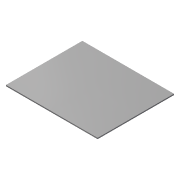
# Autodesk Inventor part: Деталь141
Saved by Autodesk Inventor 2017 (Build 210142000, 142)
## iProperties
Created: 2018-07-05
Part Number: Деталь141
Material: Сталь
Document SubType Name: Sheet Metal
Designer: Евтушенко
Mass: 6256.27 g
Surface Area: 5387.28 cm^2
Volume: 796.978 cm^3
Density: 7.85 g/cm^3
Sheet Metal Rule: ЧЗСК 1,5 мм
Appearance: Сталь
Author: Евтушенко
Autodesk Inventor part; units mm, degrees
note: some values were not read from the file. Chosen so that the rebuilt part matches the saved one: flange form of "Пластина3".
ref_plane "YZ Plane" through (0, 0, 0) normal (1, 0, 0) x (0, 1, 0)
ref_plane "XZ Plane" through (0, 0, 0) normal (0, 1, 0) x (-1, 0, 0)
ref_plane "XY Plane" through (0, 0, 0) normal (0, 0, 1) x (1, 0, 0)
sketch "Эскиз5" plane through (0, 0, 0) normal (0, 0, 1) x (1, 0, 0)
  line L0 (-60, -67.5) -> (60, -67.5)
  line L1 (60, -67.5) -> (60, 67.5)
  line L2 (60, 67.5) -> (-60, 67.5)
  line L3 (-60, 67.5) -> (-60, -67.5)
  line L4 (-60, -67.5) -> (60, 67.5) construction
  line L5 (60, -67.5) -> (-60, 67.5) construction
  point P0 (0, 0)
  dimension "d64" = 120
  dimension "d65" = 135
  measures "d64" distance of L2.end L1.end
  measures "d65" distance of L1.end L0.end
extrude "Пластина2" add sketch "Эскиз5" along normal blind 1.5
sketch "Эскиз6" plane through (-58.5, 67.5, 1.5) normal (-1, 0, 0) x (0, -1, 0)
  line L0 (135, 0) -> (0, 0)
  line L1 (0, 0) -> (0, -100)
  line L2 (0, -100) -> (135, -100)
  line L3 (135, -100) -> (135, 0)
  constraints: 6 end point, 1 horizontal, 1 perpendicular, 1 vertical
edge flange "Фланец1" height 100 angle 90 thickness 1.5 bend radius 1.1 thickness toward (-1, 0, 0) relief tear relief width 1.5 relief depth 0.75 corner gap 1.1 corner form 0 edges at (-60, 0, 0) (60, 0, 0) wall of the first edge with corners at (-58.5, -67.5, 1.5) (-58.5, 67.5, 1.5) (-58.5, 67.5, -98.5) (-58.5, -67.5, -98.5)
bend "Сгиб1"
corner "УглСтык1"
chamfer "УглФаска1" distance 35 distance2 42 1 edges at (-59.25, -67.5, -98.5) measured on face at (-59, -22.5, -98.5)
chamfer "УглФаска2" distance 42 distance2 35 1 edges at (59.25, -67.5, -98.5) measured on face at (19.1333, -67.5, 1)
equation "\"d67\" = Ширина_просечки"
equation "\"d68\" = Глубина_просечки"
equation "\"d69\" = Минимальный_остаток"
equation "\"d70\" = Радиус_гибки"
equation "\"d73\" = Радиус_гибки"
equation "\"d74\" = Размер_высечки"
equation "\"d75\" = Размер_зазора"
equation "\"d76\" = Радиус_Якоби"
equation "\"Ширина_просечки\" = Толщина"
equation "\"Глубина_просечки\" = 0.5 * Толщина"
equation "\"Размер_высечки\" = 4 * Толщина"
equation "\"Минимальный_остаток\" = 2 * Толщина"
equation "\"Радиус_перехода\" = Радиус_гибки"
equation "\"Радиус_Якоби\" = Радиус_гибки"
equation "\"Размер_зазора\" = Толщина"
equation "\"d2\" = Радиус_гибки"
equation "\"d66\" = Радиус_гибки"
equation "\"Радиус_гибки\" = 1.1"
equation "\"Толщина\" = 1.5"
